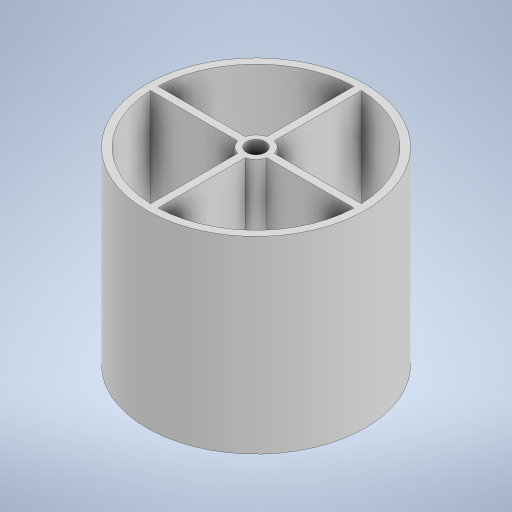
# Autodesk Inventor part: Tambor
Saved by Autodesk Inventor 2023 (Build 270158000, 158)
## iProperties
Created: 2022-11-24
Part Number: Tambor
Material: Genérico
Document SubType Name: Modeling
Designer: sergi
Density: 1 g/cm^3
Appearance: Valor por defecto
Author: sergi
Autodesk Inventor part; units mm, degrees
ref_plane "YZ Plane" through (0, 0, 0) normal (1, 0, 0) x (0, 1, 0)
ref_plane "XZ Plane" through (0, 0, 0) normal (0, 1, 0) x (-1, 0, 0)
ref_plane "XY Plane" through (0, 0, 0) normal (0, 0, 1) x (1, 0, 0)
sketch "Boceto1" plane through (0, 0, 0) normal (0, 1, 0) x (-1, 0, 0)
  circle A0 centre (0, 0) radius 29
  dimension "d0" = 58
  constraints: 1 centre point, 1 coincident
  measures "d0" diameter of A0
extrude "Extrusión1" add sketch "Boceto1" along normal blind 50
shell "Vaciado1" thickness 2 removed faces 2 at (2.104, 0, -7.1206) at (2.104, 50, -7.1206)
sketch "Boceto2" plane through (0, 0, 0) normal (0, -1, 0) x (1, 0, 0)
  line L0 (1, 28.5) -> (-1, 28.5)
  line L1 (-1, -28.5) -> (1, -28.5)
  line L2 (-28.5, 1) -> (-28.5, -1)
  line L3 (28.5, -1) -> (28.5, 1)
  line L4 (-19.4454, 20.8597) -> (-20.8597, 19.4454)
  line L5 (19.4454, -20.8597) -> (20.8597, -19.4454)
  line L6 (-64.7852, 95.7171) -> (-23.0659, 56.8262) construction
  line L7 (-20.8597, -19.4454) -> (-19.4454, -20.8597)
  line L8 (20.8597, 19.4454) -> (19.4454, 20.8597)
  arc A0 (-1, 3.873) -> (-2.0315, 3.4457) centre (0, 0) ccw
  line L9 (-1, 28.5) -> (-1, 3.873)
  line L10 (-3.873, 1) -> (-28.5, 1)
  line L11 (-28.5, -1) -> (-3.873, -1)
  line L12 (3.873, -1) -> (28.5, -1)
  line L13 (28.5, 1) -> (3.873, 1)
  line L14 (-1, -3.873) -> (-1, -28.5)
  line L15 (1, -28.5) -> (1, -3.873)
  line L16 (1, 3.873) -> (1, 28.5)
  arc A1 (3.873, 1) -> (1, 3.873) centre (0, 0) ccw
  arc A2 (1, -3.873) -> (3.873, -1) centre (0, 0) ccw
  arc A3 (1, -3.873) -> (3.873, -1) centre (0, 0) ccw
  arc A4 (-3.873, -1) -> (-1, -3.873) centre (0, 0) ccw
  arc A5 (-3.873, -1) -> (-1, -3.873) centre (0, 0) ccw
  arc A6 (-3.4457, 2.0315) -> (-3.873, 1) centre (0, 0) ccw
  arc A7 (3.873, 1) -> (1, 3.873) centre (0, 0) ccw
  arc A8 (-1, 3.873) -> (-3.873, 1) centre (0, 0) ccw
  circle A9 centre (0, 0) radius 2.5
  dimension "d4" = 2
  dimension "d5" = 57
  dimension "d6" = 57
  dimension "d7" = 2
  dimension "d12" = 2
  dimension "d13" = 57
  dimension "d14" = 57
  dimension "d15" = 2
  dimension "d17" = 5
  constraints: 34 end point, 19 point on circle, 12 parallel, 10 centre point, 4 perpendicular, 3 horizontal, 1 coincident
  measures "d4" distance of L1.end L1.start
  measures "d5" distance of L1.start L0.end
  measures "d6" distance of L3.start L2.end
  measures "d7" distance of L2.end L2.start
  measures "d12" distance of L5.end L5.start
  measures "d13" distance of L5.start L4.end
  measures "d14" distance of L8.start L7.end
  measures "d15" distance of L7.end L7.start
  measures "d17" diameter of A9
extrude "Extrusión2" add sketch "Boceto2" against normal blind 50
